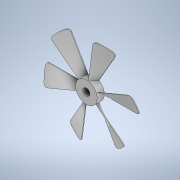
# Autodesk Inventor part: Fan
Saved by Autodesk Inventor 2022 (Build 260153000, 153)
## iProperties
Created: 2021-07-24
Part Number: Fan
Material: Generic
Document SubType Name: Modeling
Designer: Mike
Density: 1 g/cm^3
Appearance: Default
Author: Mike
Autodesk Inventor part; units mm, degrees
ref_plane "YZ Plane" through (0, 0, 0) normal (1, 0, 0) x (0, 1, 0)
ref_plane "XZ Plane" through (0, 0, 0) normal (0, 1, 0) x (-1, 0, 0)
ref_plane "XY Plane" through (0, 0, 0) normal (0, 0, 1) x (1, 0, 0)
sketch "Sketch1" plane through (0, 0, 0) normal (0, 0, 1) x (1, 0, 0)
  circle A0 centre (0, 0) radius 7.5
  circle A1 centre (0, 0) radius 2.5
  dimension "d0" = 15
  dimension "d1" = 5
  constraints: 2 centre point, 2 coincident
  measures "d0" diameter of A0
  measures "d1" diameter of A1
extrude "Extrusion1" add sketch "Sketch1" against normal blind 5
sketch "Sketch3" plane through (0, 0, 0) normal (0, 1, 0) x (-1, 0, 0)
  line L0 (-7.5, -5) -> (7.5, -5) projected
  line L1 (-7.5, -5) -> (-32.5, -5)
  line L2 (-32.5, -5) -> (-32.5, -4.5)
  line L3 (-32.5, -4.5) -> (-7.5, -4.5)
  line L4 (-7.5, -4.5) -> (-7.5, -5)
  point P0 (0, 0)
  dimension "d5" = 0.5
  dimension "d6" = 25
  constraints: 8 end point, 2 parallel, 1 horizontal, 1 perpendicular
  measures "d5" distance between parallel lines of L3 L1
  measures "d6" distance between parallel lines of L2 L4
coil "Coil1" sketch "Sketch3" operation add axis through (0, 0, -10) along (0, 0, 1) pitch 63.4921 turns 0.063 hand right
fillet "Fillet1" radius 2 2 edges at (29.9869, 12.5315, -0.75) (32.5, 0, -4.75)
pattern_circular "Circular Pattern1" count 6 over 360 about axis through (0, 0, -10) along (0, 0, 1) of "Coil1", "Fillet1"
body "Solid1"
